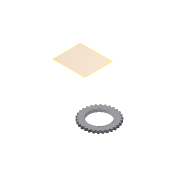
# Autodesk Inventor part: 30_Nut_Gear
Saved by Autodesk Inventor 2016 (Build 200138000, 138)
## iProperties
Created: 2016-12-20
Part Number: 30_Nut_Gear
Material: Generisch
Document SubType Name: Modeling
Designer: diederichbenedict
Density: 1 g/cm^3
Appearance: Vorgabe
Author: diederichbenedict
Autodesk Inventor part; units mm, degrees
ref_plane "YZ Plane" through (0, 0, 0) normal (1, 0, 0) x (0, 1, 0)
ref_plane "XZ Plane" through (0, 0, 0) normal (0, 1, 0) x (-1, 0, 0)
ref_plane "XY Plane" through (0, 0, 0) normal (0, 0, 1) x (1, 0, 0)
ref_plane "Arbeitsebene1" through (-99.9683, 72.359, 0) normal (0, 0, 1) x (1, 0.0059, 0)
sketch "Skizze1" plane through (-99.9683, 72.359, 0) normal (0, 0, 1) x (1, 0.0059, 0)
  line L0 (111.9405, -52.0134) -> (123.9403, -73.0848) construction
  line L1 (87.6922, -51.8699) -> (111.9405, -52.0134) construction
  line L2 (75.4438, -72.7978) -> (87.6922, -51.8699) construction
  line L3 (87.4437, -93.8692) -> (75.4438, -72.7978) construction
  line L4 (111.6919, -94.0127) -> (87.4437, -93.8692) construction
  line L5 (123.9403, -73.0848) -> (111.6919, -94.0127) construction
  circle A0 centre (99.6921, -72.9413) radius 18.5 construction
  line L6 (87.9779, -52.3716) -> (111.6488, -52.5117)
  line L7 (111.6488, -52.5117) -> (123.363, -73.0814)
  line L8 (123.363, -73.0814) -> (111.4062, -93.511)
  line L9 (111.4062, -93.511) -> (87.7353, -93.3709)
  line L10 (87.7353, -93.3709) -> (76.0211, -72.8013)
  line L11 (76.0211, -72.8013) -> (87.9779, -52.3716)
  circle A1 centre (99.6921, -72.9413) radius 18.75
  circle A2 centre (99.6921, -72.9413) radius 17.5 projected
  circle A3 centre (99.6921, -72.9413) radius 18
  circle A4 centre (99.6921, -73.0848) radius 23.7953
  point P0 (99.5384, -72.9493)
  dimension "d0" = 0.5
  dimension "d1" = 0.25
  dimension "d4" = 0.5
  constraints: 12 end point, 2 centre point, 8 other
  measures "d0" distance between parallel lines of L2 L11
  measures "d1" radial gap between concentric circles of A0 A1
  measures "d4" radial gap between concentric circles of A2 A3
extrude "Extrusion1" add sketch "Skizze1" along normal blind 4 contours A4 L6 | L6 L7 L8 L9 L10 L11 | L11 L10 L9 L8 L7 A4 | A1
thread "Gewinde1" size "M36x1.5" class "6H" standard "ANSI Metric M Profile" full length
sketch "Skizze3" plane through (0, 0, 4) normal (-1, 0, 0) x (0, 1, 0)
  line L0 (18.0089, 0) -> (18.0089, 4)
  line L1 (18.0089, 4) -> (16.9962, 4)
  line L2 (16.9962, 4) -> (16.9962, 0)
  line L3 (16.9962, 0) -> (18.0089, 0)
  line L4 (0, -17.9216) -> (0, 25.8821)
  line L5 (18.0089, 4) -> (18.0089, 0)
  spline S0 degree 3 number of poles 544 construction
  constraints: 8 end point, 1 point on line
revolve "Umdrehung1" add sketch "Skizze3" angle 360 about axis through (0, 0, 4) along (0, 0, -1) separate body
sketch "Skizze2" plane through (0, 17.25, 4) normal (1, 0, 0) x (0, 0, -1)
  line L0 (-2.6757, 0.5451) -> (-2.537, 0.5451) construction
  line L1 (-1.6484, -0.2737) -> (-1.787, -0.5138) construction
  line L2 (-3.287, -0.5138) -> (-3.4257, -0.2737) construction
  line L3 (-2.3984, 0.5451) -> (-2.537, 0.7852) construction
  line L4 (-2.537, 0.7852) -> (-2.6757, 0.5451) construction
  line L5 (-3.287, -0.5138) -> (-3.1484, -0.2737) construction
  line L6 (-2.3984, 0.5451) -> (-1.9257, -0.2737)
  line L7 (-3.4257, -0.2737) -> (-3.1484, -0.2737) construction
  arc A0 (-3.4257, -0.2737) -> (-3.287, -0.3538) centre (-3.287, -0.1937) ccw construction
  line L8 (-1.6484, -0.2737) -> (-1.9257, -0.2737) construction
  line L9 (-3.287, -0.5138) -> (-3.287, -0.2737) construction
  line L10 (-1.787, -0.5138) -> (-1.787, -0.2737) construction
  line L11 (-2.537, 0.7852) -> (-2.537, 0.6251) construction
  line L12 (-3.287, -0.3538) -> (-1.787, -0.3538)
  arc A1 (-3.287, -0.3538) -> (-3.1484, -0.2737) centre (-3.287, -0.1937) ccw
  line L13 (-1.9257, -0.2737) -> (-1.787, -0.5138) construction
  line L14 (-3.1484, -0.2737) -> (-2.6757, 0.5451)
  line L15 (-1.787, 0.6251) -> (-1.787, 0.3871)
  line L16 (-1.787, 0.3871) -> (-1.787, 0.6251)
  line L17 (-1.787, 0.6251) -> (-1.7535, 0.6251)
  arc A2 (-1.9257, -0.2737) -> (-1.787, -0.3538) centre (-1.787, -0.1937) ccw
  arc A3 (-1.787, -0.3538) -> (-1.6484, -0.2737) centre (-1.787, -0.1937) ccw construction
  arc A4 (-2.537, 0.6251) -> (-2.6757, 0.5451) centre (-2.537, 0.465) ccw
  arc A5 (-2.3984, 0.5451) -> (-2.537, 0.6251) centre (-2.537, 0.465) ccw
  line L18 (-2.537, 0.6251) -> (-2.537, 0.5451) construction
  line L19 (-2.537, 0.5451) -> (-2.3984, 0.5451) construction
  line L20 (4, 0.7589) -> (0, 0.7589) projected
  line L21 (4, -0.2538) -> (0, -0.2538) projected
  dimension "d8" = 60
  dimension "d9" = 0.2401
  dimension "d10" = 0.2401
  dimension "Skizze2_ThreadOffset" = 0
  dimension "Skizze2_MajorRadius" = 0.9789
  dimension "d13" = 1.5
  dimension "Skizze2_MinorRadius" = 0
  dimension "d27" = 0.1
  constraints: 40 end point, 12 point on circle, 10 parallel, 8 tangent, 6 centre point, 6 collinear, 2 midpoint, 2 point on line, 1 horizontal, 1 perpendicular
  measures "d8" angle of L6 L14
  measures "d9" distance of L3.end L0.end
  measures "d10" distance of L1.end L10.end
  measures "Skizze2_ThreadOffset" distance between parallel lines of L15 L10
  measures "Skizze2_MajorRadius" distance from line of L12 L15.start
  measures "d13" distance from line of L1.end L9
  measures "Skizze2_MinorRadius" distance edge to line of A5 L17
  measures "d27" distance between parallel lines of L21 L12
coil "Spirale1" sketch "Skizze2" operation cut axis through (0, 0, 4) along (0, 0, -1) pitch 1.5015 turns 4.662005 hand right bodies 2
sketch "Skizze4" plane through (0.1545, -0.1346, 4) normal (0, 0, 1) x (1, 0, 0)
  line L0 (-0.1545, 0.1346) -> (28, 0.1346) construction
  circle A0 centre (-0.0008, 0.1435) radius 18 construction
  arc A1 (28, 0.1346) -> (23.5883, 3.1318) centre (21.1448, -5.2105) ccw
  circle A2 centre (0, 0) radius 23.7953 projected
  arc A3 (23.5883, -2.8626) -> (28, 0.1346) centre (21.1448, 5.4797) ccw
  line L1 (23.5883, 3.1318) -> (23.5883, -2.8626)
  constraints: 4 end point, 4 point on circle, 2 centre point, 2 coincident, 2 symmetric about line, 1 horizontal, 1 vertical, 3 other
extrude "Extrusion2" add sketch "Skizze4" against normal up to surface (4 mm away) contours A3 A2 A1 | A2 A3 L1 picked at (23.6266, 0.7868) bodies 1
pattern_circular "Runde Anordnung1" count 30 over 360 about axis through (0.1536, 0.0089, 0) along (0, 0, 1) of "Extrusion2" bodies 1
equation "\"d8\" = d15"
equation "\"d9\" = 0.160083 * Skizze2_Pitch"
equation "\"d10\" = 0.160083 * Skizze2_Pitch"
equation "\"d13\" = Skizze2_Pitch"
equation "\"d15\" = 60deg"
equation "\"Skizze2_Pitch\" = 1.5"
